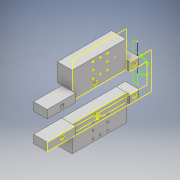
# Autodesk Inventor part: support_arret
Saved by Autodesk Inventor 2017 (Build 210142000, 142)
## iProperties
Part Number: support_arret
Material: Générique
Document SubType Name: Modeling
Designer: Thomas
Density: 1 g/cm^3
Appearance: Par défaut
Author: Thomas
Autodesk Inventor part; units mm, degrees
ref_plane "YZ Plane" through (0, 0, 0) normal (1, 0, 0) x (0, 1, 0)
ref_plane "XZ Plane" through (0, 0, 0) normal (0, 1, 0) x (-1, 0, 0)
ref_plane "XY Plane" through (0, 0, 0) normal (0, 0, 1) x (1, 0, 0)
sketch "Esquisse1" plane through (0, 0, 0) normal (1, 0, 0) x (0, 1, 0)
  line L0 (-54.8063, -40.1439) -> (54.7548, -40.1439)
  line L1 (54.7548, 0.0046) -> (-54.8063, 0.0046)
  line L2 (41.6156, -39.9954) -> (41.6156, -34.9954) construction
  line L3 (41.6156, -34.9954) -> (-43.4679, -34.9954) construction
  circle A0 centre (41.6156, -34.9954) radius 2.15
  circle A1 centre (1.6156, -34.9954) radius 2.15
  circle A2 centre (-38.3844, -34.9954) radius 2.15
  circle A3 centre (41.6156, -4.9954) radius 2.15
  circle A4 centre (1.6156, -4.9954) radius 2.15
  circle A5 centre (-38.3844, -4.9954) radius 2.15
  line L4 (-38.3844, 0.0046) -> (-38.3844, -4.9954) construction
  line L5 (54.7548, -40.1439) -> (59.7548, -40.1439)
  line L6 (59.7548, -40.1439) -> (59.7548, 0.0046)
  line L7 (59.7548, 0.0046) -> (54.7548, 0.0046)
  line L8 (-54.8063, -31.1439) -> (55.1937, -31.1439)
  line L9 (-54.8063, -8.9954) -> (55.1937, -8.9954)
  line L10 (-54.8063, 0.0046) -> (-54.8063, -8.9954)
  line L11 (-54.8063, -31.1439) -> (-54.8063, -40.1439)
  line L12 (55.1937, -31.1439) -> (55.1937, -8.9954)
  line L13 (-54.8063, -31.1439) -> (-54.8063, -40.1439)
  line L14 (-54.8063, -40.1439) -> (59.7548, -40.1439)
  line L15 (59.7548, -40.1439) -> (59.7548, 0.0046)
  line L16 (59.7548, 0.0046) -> (-54.8063, 0.0046)
  line L17 (-54.8063, 0.0046) -> (-54.8063, -8.9954)
  line L18 (-54.8063, -8.9954) -> (55.1937, -8.9954)
  line L19 (55.1937, -8.9954) -> (55.1937, -31.1439)
  line L20 (55.1937, -31.1439) -> (-54.8063, -31.1439)
  point P0 (0, 0)
  point P1 (60.2697, -11.7227)
  dimension "d4" = 5
  dimension "d5" = 4.3
  dimension "d6" = 40
  dimension "d7" = 30
  dimension "d8" = 5
  dimension "d9" = 5
  dimension "d10" = 110
  dimension "d11" = 9
  dimension "d12" = 110
  dimension "d14" = 40.1485
  dimension "d15" = 9
  constraints: 42 end point, 6 centre point, 5 collinear, 5 horizontal, 4 perpendicular, 4 vertical, 2 coincident, 2 parallel, 1 point on line, 10 other
  measures "d4" distance of L2.start L2.end
  measures "d5" diameter of A0
  measures "d6" distance of A0.centre A1.centre
  measures "d7" distance of A0.centre A3.centre
  measures "d8" distance of L4.start L4.end
  measures "d9" distance of L7.end L6.end
  measures "d10" distance of L8.start L8.end
  measures "d11" distance between parallel lines of L8 L0
  measures "d12" distance of L9.start L9.end
  measures "d14" distance between parallel lines of L1 L0
  measures "d15" distance between parallel lines of L1 L9
extrude "Extrusion1" add sketch "Esquisse1" along normal blind 15
sketch "Esquisse2" plane through (0, 59.7548, 0.0046) normal (0, 1, 0) x (1, 0, 0)
  point P0 (0, 0.0046)
sketch "Esquisse3" plane through (0, 59.7548, 0.0046) normal (0, 1, 0) x (1, 0, 0)
  line L0 (-4.433, 21.1485) -> (-2.433, 21.1485)
  arc A0 (11.3752, 24.099) -> (-2.433, 21.1485) centre (5, 20.1485) ccw
  line L1 (11.3752, 24.099) -> (12.5262, 24.099)
  arc A1 (12.5262, 24.099) -> (5, 28.6485) centre (5, 20.1485) ccw
  line L2 (5, 28.6485) -> (5, 30.0821)
  line L3 (5, 30.0821) -> (0, 30.0821)
  line L4 (0, 30.0821) -> (0, 40.1485)
  line L5 (-5.0769, 40.1485) -> (0, 40.1485)
  line L6 (-5.0769, 0.1485) -> (-5.0769, 40.1485)
  line L7 (0, 0.1485) -> (-5.0769, 0.1485)
  line L8 (0, 10.1485) -> (0, 0.1485)
  line L9 (0, 10.1485) -> (5, 10.1485)
  line L10 (5, 10.1485) -> (5, 11.6485)
  arc A2 (5, 11.6485) -> (12.5262, 16.1979) centre (5, 20.1485) ccw
  line L11 (12.5262, 16.1979) -> (11.3752, 16.1979)
  arc A3 (-2.433, 19.1485) -> (11.3752, 16.1979) centre (5, 20.1485) ccw
  line L12 (-2.433, 19.1485) -> (-4.433, 19.1485)
  line L13 (-4.433, 19.1485) -> (-4.433, 21.1485)
  line L14 (0, 0) -> (0, 9) projected
  line L15 (0, 40.1485) -> (0, 0)
  point P0 (0, 0.0046)
  point P1 (-5.0769, 30.0821)
  constraints: 30 end point, 8 point on circle, 4 centre point, 2 collinear
sketch "Esquisse4" plane through (0, 59.7548, 0.0046) normal (0, 1, 0) x (1, 0, 0)
  circle A0 centre (5.0199, 20.1961) radius 6
  circle A1 centre (5.0199, 20.1961) radius 6
  point P0 (0, 0.0046)
  dimension "d18" = 12
  constraints: 2 centre point, 1 coincident, 1 concentric
  measures "d18" diameter of A0
extrude "Extrusion2" cut sketch "Esquisse4" against normal blind 15
sketch "Esquisse5" plane through (0, -54.8063, 0.0046) normal (0, 0, 1) x (1, 0, 0)
  line L0 (15, 114.5611) -> (15, 0) construction
  line L1 (15, 114.5611) -> (11.2, 114.5611) construction
  line L2 (0, 114.5611) -> (15, 114.5611) construction
  line L3 (11.2, 114.5611) -> (11.2, 58.3541) construction
  line L4 (15, 91.0895) -> (11.2, 91.0895)
  line L5 (11.2, 91.0895) -> (11.2, 31.0895)
  line L6 (11.2, 31.0895) -> (15, 31.0895)
  line L7 (15, 31.0895) -> (15, 91.0895)
  point P0 (0, 54.8063)
  dimension "d21" = 3.8
  dimension "d22" = 60
  constraints: 12 end point, 4 perpendicular, 4 point on line, 1 collinear
  measures "d21" distance of L0.start L1.end
  measures "d22" distance of L4.end L5.end
extrude "Extrusion3" cut sketch "Esquisse5" against normal blind 15
sketch "Esquisse6" plane through (0, -54.8063, 0.0046) normal (0, 0, 1) x (1, 0, 0)
  line L0 (11.2, 91.0895) -> (11.2, 31.0895) projected
  line L1 (11.2, 91.0895) -> (-5, 91.0895)
  line L2 (-5, 91.0895) -> (-5, 31.3621)
  line L3 (-5, 31.3621) -> (11.2, 31.3621)
  line L4 (11.2, 31.3621) -> (11.2, 91.0895)
  point P0 (0, 54.8063)
  dimension "d25" = 16.2
  constraints: 8 end point, 2 parallel, 1 horizontal, 1 perpendicular
  measures "d25" distance of L3.end L2.end
extrude "Extrusion4" add sketch "Esquisse6" along normal blind 30
sketch "Esquisse7" plane through (11.2, -23.7168, -8.9954) normal (1, 0, 0) x (0, 0, -1)
  line L0 (0, 60) -> (0, 0) projected
  line L1 (-9, 60) -> (0, 60) projected
  line L2 (-9, 60) -> (-39, 60) projected
  line L3 (-39, 0.2726) -> (-39, 60) projected
  line L4 (-9, 0.2726) -> (-39, 0.2726) projected
  line L5 (-9, 0) -> (-9, 0.2726) projected
  line L6 (-9, 0) -> (0, 0) projected
  circle A0 centre (-4, 25.3324) radius 2.15 projected
  circle A1 centre (-10, 31.1304) radius 1
  circle A2 centre (-18, 39.1304) radius 1
  circle A3 centre (-26, 39.1304) radius 1
  circle A4 centre (-26, 31.1304) radius 1
  circle A5 centre (-26, 23.1304) radius 1
  circle A6 centre (-18, 23.1304) radius 1
  circle A7 centre (-10, 23.1304) radius 1
  circle A8 centre (-10, 39.1304) radius 1
  point P0 (-8.9954, 23.7168)
  dimension "d28" = 10
  dimension "d29" = 16
  dimension "d30" = 8
  dimension "d31" = 8
  dimension "d32" = 8
  dimension "d33" = 8
  dimension "d34" = 8
  dimension "d35" = 8
  constraints: 8 centre point
  measures "d28" distance from line of L0 A1.centre
  measures "d29" distance of A4.centre A1.centre
  measures "d30" distance of A7.centre A1.centre
  measures "d31" distance of A8.centre A1.centre
  measures "d32" distance of A6.centre A7.centre
  measures "d33" distance of A5.centre A6.centre
  measures "d34" distance of A2.centre A8.centre
  measures "d35" distance of A3.centre A2.centre
extrude "Extrusion5" cut sketch "Esquisse7" against normal blind 30 contours A1 | A2 | A3 | A4 | A5 | A6 | A7 | A8
sketch "Esquisse8" plane through (15, 0, 0) normal (1, 0, 0) x (0, 0, -1)
  line L0 (-0.0046, 36.2832) -> (8.9954, 36.2832) projected
  line L1 (8.9954, 36.2832) -> (8.9954, 55.1937) projected
  line L2 (8.9954, 55.1937) -> (31.1439, 55.1937) projected
  line L3 (31.1439, 55.1937) -> (31.1439, -54.8063) projected
  line L4 (31.1439, -54.8063) -> (40.1439, -54.8063) projected
  line L5 (40.1439, -54.8063) -> (40.1439, 59.7548) projected
  line L6 (40.1439, 59.7548) -> (-0.0046, 59.7548) projected
  line L7 (-0.0046, 59.7548) -> (-0.0046, 36.2832) projected
  circle A0 centre (4.9954, 41.6156) radius 2.15 projected
  circle A1 centre (34.9954, -38.3844) radius 2.15 projected
  circle A2 centre (34.9954, 1.6156) radius 2.15 projected
  circle A3 centre (34.9954, 41.6156) radius 2.15 projected
  point P0 (0, 0)
sketch "Esquisse9" plane through (11.2, -23.7168, -8.9954) normal (1, 0, 0) x (0, 0, -1)
  circle A0 centre (-10, 23.1304) radius 1 projected
  circle A1 centre (-26, 23.1304) radius 1 projected
  circle A2 centre (-26, 39.1304) radius 1 projected
  circle A3 centre (-10, 31.1304) radius 1 projected
  circle A4 centre (-18, 39.1304) radius 1 projected
  circle A5 centre (-26, 31.1304) radius 1 projected
  circle A6 centre (-18, 23.1304) radius 1 projected
  circle A7 centre (-10, 39.1304) radius 1 projected
  line L0 (0, 60) -> (0, 0) projected
  line L1 (-9, 60) -> (0, 60) projected
  line L2 (-9, 60) -> (-39, 60) projected
  line L3 (-39, 0.2726) -> (-39, 60) projected
  line L4 (-9, 0.2726) -> (-39, 0.2726) projected
  line L5 (-9, 0) -> (-9, 0.2726) projected
  line L6 (-9, 0) -> (0, 0) projected
  circle A8 centre (-4, 25.3324) radius 2.15 projected
  point P0 (-8.9954, 23.7168)
sketch "Esquisse10" plane through (15, 0, 0) normal (1, 0, 0) x (0, 0, -1)
  line L0 (31.0084, 36.2646) -> (31.0084, -23.7354)
  circle A0 centre (41.0084, -0.605) radius 1
  circle A1 centre (57.0084, -0.605) radius 1
  circle A2 centre (57.0084, 15.395) radius 1
  circle A3 centre (41.0084, 7.395) radius 1
  circle A4 centre (49.0084, 15.395) radius 1
  circle A5 centre (57.0084, 7.395) radius 1
  circle A6 centre (49.0084, -0.605) radius 1
  circle A7 centre (41.0084, 15.395) radius 1
  line L1 (40.0084, 36.2646) -> (31.0084, 36.2646)
  line L2 (40.0084, 36.2646) -> (70.0084, 36.2646)
  line L3 (70.0084, -23.4628) -> (70.0084, 36.2646)
  line L4 (40.0084, -23.4628) -> (70.0084, -23.4628)
  line L5 (40.0084, -23.7354) -> (40.0084, -23.4628)
  line L6 (40.0084, -23.7354) -> (31.0084, -23.7354)
  circle A8 centre (35.0084, 1.597) radius 2.15
  point P0 (0, 0)
  point P1 (40.0039, -0.0185)
  constraints: 14 end point, 9 centre point
extrude "Extrusion6" cut sketch "Esquisse10" against normal blind 3.8 contours L1 L2 L3 L4 L5 L6 L0 | A0 | A1 | A2 | A3 | A4 | A5 | A6 | A7 | A8
sketch "Esquisse11" plane through (11.2, 0, 0) normal (1, 0, 0) x (0, 0, -1)
  circle A0 centre (34.9954, 1.6156) radius 2.15 projected
  line L0 (31.1439, -23.7354) -> (31.1439, 36.2646) projected
  line L1 (40.0084, -23.7354) -> (31.1439, -23.7354) projected
  line L2 (40.0084, -23.4628) -> (40.0084, -23.7354) projected
  line L3 (40.1439, -23.4628) -> (40.0084, -23.4628) projected
  line L4 (40.1439, 36.2646) -> (40.1439, -23.4628) projected
  line L5 (31.1439, 36.2646) -> (40.1439, 36.2646) projected
  point P0 (0, 0)
sketch "Esquisse12" plane through (11.2, 0, 0) normal (1, 0, 0) x (0, 0, -1)
  point P0 (-8.9954, 23.7168)
sketch "Esquisse13" plane through (11.2, 0, 0) normal (1, 0, 0) x (0, 0, -1)
  line L0 (30.9931, 36.2812) -> (30.9931, -23.7188)
  circle A0 centre (40.9931, -0.5884) radius 1
  circle A1 centre (56.9931, -0.5884) radius 1
  circle A2 centre (56.9931, 15.4116) radius 1
  circle A3 centre (40.9931, 7.4116) radius 1
  circle A4 centre (48.9931, 15.4116) radius 1
  circle A5 centre (56.9931, 7.4116) radius 1
  circle A6 centre (48.9931, -0.5884) radius 1
  circle A7 centre (40.9931, 15.4116) radius 1
  line L1 (39.9931, 36.2812) -> (30.9931, 36.2812)
  line L2 (39.9931, 36.2812) -> (69.9931, 36.2812)
  line L3 (69.9931, -23.4462) -> (69.9931, 36.2812)
  line L4 (39.9931, -23.4462) -> (69.9931, -23.4462)
  line L5 (39.9931, -23.7188) -> (39.9931, -23.4462)
  line L6 (39.9931, -23.7188) -> (30.9931, -23.7188)
  circle A8 centre (34.9931, 1.6136) radius 2.15
  point P0 (0, 0)
  point P1 (39.9885, -0.002)
  constraints: 14 end point, 9 centre point
extrude "Extrusion7" add sketch "Esquisse13" against normal blind 16.2
sketch "Esquisse14" plane through (-5, 0, 0) normal (-1, 0, 0) x (0, 0, 1)
  circle A0 centre (-56.9931, -0.5884) radius 1 projected
  circle A1 centre (-56.9931, 7.4116) radius 1 projected
  circle A2 centre (-56.9931, 15.4116) radius 1 projected
  circle A3 centre (-48.9931, 15.4116) radius 1 projected
  circle A4 centre (-48.9931, -0.5884) radius 1 projected
  circle A5 centre (-40.9931, -0.5884) radius 1 projected
  circle A6 centre (-40.9931, 7.4116) radius 1 projected
  circle A7 centre (-40.9931, 15.4116) radius 1 projected
  circle A8 centre (-56.9931, -0.5884) radius 1 projected
  circle A9 centre (-56.9931, -0.5884) radius 3
  line L0 (-56.9931, -0.5884) -> (-56.9931, 15.4116) construction
  line L1 (-56.9931, 15.4116) -> (-40.9931, 15.4116) construction
  circle A10 centre (-56.9931, 7.4116) radius 3
  circle A11 centre (-56.9931, 15.4116) radius 3
  circle A12 centre (-48.9931, -0.5884) radius 3
  circle A13 centre (-48.9931, 7.4116) radius 3
  circle A14 centre (-48.9931, 15.4116) radius 3
  circle A15 centre (-40.9931, -0.5884) radius 3
  circle A16 centre (-40.9931, 7.4116) radius 3
  circle A17 centre (-40.9931, 15.4116) radius 3
  line L2 (-26.1915, 59.7548) -> (-14.1915, 59.7548) construction
  line L3 (-20.1915, 59.7548) -> (-20.1915, -51.3949) construction
  circle A18 centre (16.6101, -0.5884) radius 1
  circle A19 centre (16.6101, 7.4116) radius 1
  circle A20 centre (16.6101, 15.4116) radius 1
  circle A21 centre (8.6101, 15.4116) radius 1
  circle A22 centre (8.6101, -0.5884) radius 1
  circle A23 centre (0.6101, -0.5884) radius 1
  circle A24 centre (0.6101, 7.4116) radius 1
  circle A25 centre (0.6101, 15.4116) radius 1
  circle A26 centre (16.6101, -0.5884) radius 1
  circle A27 centre (16.6101, -0.5884) radius 3
  line L4 (16.6101, -0.5884) -> (16.6101, 15.4116) construction
  line L5 (16.6101, 15.4116) -> (0.6101, 15.4116) construction
  circle A28 centre (16.6101, 7.4116) radius 3
  circle A29 centre (16.6101, 15.4116) radius 3
  circle A30 centre (8.6101, -0.5884) radius 3
  circle A31 centre (8.6101, 7.4116) radius 3
  circle A32 centre (8.6101, 15.4116) radius 3
  circle A33 centre (0.6101, -0.5884) radius 3
  circle A34 centre (0.6101, 7.4116) radius 3
  circle A35 centre (0.6101, 15.4116) radius 3
  point P0 (0, 0)
  point P1 (-23.478, 59.7548)
  point P2 (-16.9051, 59.7548)
  dimension "d44" = 6
  dimension "d47" = 8
  dimension "d50" = 8
  constraints: 27 centre point, 18 symmetric about line, 10 end point, 3 vertical, 2 coincident, 1 horizontal, 1 midpoint, 1 perpendicular, 34 other
  measures "d44" diameter of A9
  measures "d47" distance of A9.centre A10.centre
  measures "d50" distance of A9.centre A12.centre
extrude "Extrusion8" cut sketch "Esquisse14" against normal blind 8 contours A0 | A1 | A2 | A3 | A4 | A5 | A6 | A7 | A9 | A10 | A11 | A12 | A14 | A15 | A16 | A17 | A18 | A19 | A20 | A21 | A22 | A23 | A24 | A25 | A27 | A28 | A29 | A30 | A32 | A33 | A34 | A35
sketch "Esquisse15" plane through (-5, 0, 0) normal (-1, 0, 0) x (0, 0, 1)
  line L0 (-39.9931, -23.7188) -> (-30.9931, -23.7188) projected
  line L1 (-40.1439, 36.2646) -> (-40.1439, 59.7548) projected
  line L2 (-30.9931, -23.7188) -> (-40.1439, -23.7188)
  line L3 (-40.1439, -23.7188) -> (-40.1439, 36.2646)
  line L4 (-40.1439, 36.2646) -> (-30.9931, 36.2646)
  line L5 (-30.9931, 36.2646) -> (-30.9931, -23.7188)
  line L6 (-40.1439, 36.2646) -> (-30.9931, 36.2646)
  line L7 (-30.9931, 36.2646) -> (-30.9931, 36.6984)
  line L8 (-30.9931, 36.6984) -> (-40.1439, 36.6984)
  line L9 (-40.1439, 36.6984) -> (-40.1439, 36.2646)
  point P0 (0, 0)
  constraints: 16 end point, 4 parallel, 2 horizontal, 2 perpendicular
extrude "Extrusion9" cut sketch "Esquisse15" against normal blind 5
sketch "Esquisse16" plane through (11.2, -23.7188, -30.9931) normal (0, 0, 1) x (1, 0, 0)
  line L0 (-11.2, 60) -> (-11.2, 0) projected
  line L1 (0, 0) -> (-11.2, 0) projected
  line L2 (0, 0) -> (0, 60) projected
  line L3 (0, 60) -> (-11.2, 60) projected
  point P0 (-11.2, 23.7188)
extrude "Extrusion10" cut sketch "Esquisse16" against normal blind 0.15
sketch "Esquisse17" plane through (11.2, 0, 0) normal (1, 0, 0) x (0, 0, -1)
  line L0 (31.1431, 36.2812) -> (31.1431, -23.7188) projected
  line L1 (31.1439, -23.7188) -> (31.1431, -23.7188) projected
  line L2 (31.1439, -23.7354) -> (31.1439, -23.7188) projected
  line L3 (40.0084, -23.7354) -> (31.1439, -23.7354) projected
  line L4 (40.0084, -23.4628) -> (40.0084, -23.7354) projected
  line L5 (40.1439, -23.4628) -> (40.0084, -23.4628) projected
  line L6 (40.1439, -23.4462) -> (40.1439, -23.4628) projected
  line L7 (69.9931, -23.4462) -> (40.1439, -23.4462) projected
  line L8 (69.9931, 36.2812) -> (69.9931, -23.4462) projected
  line L9 (40.1439, 36.2812) -> (69.9931, 36.2812) projected
  line L10 (40.1439, 36.2646) -> (40.1439, 36.2812) projected
  line L11 (31.1439, 36.2646) -> (40.1439, 36.2646) projected
  line L12 (31.1439, 36.2812) -> (31.1439, 36.2646) projected
  line L13 (31.1431, 36.2812) -> (31.1439, 36.2812) projected
  line L14 (40.1439, -0.0603) -> (40.1439, -1.1165) projected
  arc A0 (40.1439, -1.1165) -> (40.1439, -0.0603) centre (40.9931, -0.5884) ccw projected
  line L15 (40.1439, 7.9397) -> (40.1439, 6.8835) projected
  arc A1 (40.1439, 6.8835) -> (40.1439, 7.9397) centre (40.9931, 7.4116) ccw projected
  line L16 (40.1439, 15.9397) -> (40.1439, 14.8835) projected
  arc A2 (40.1439, 14.8835) -> (40.1439, 15.9397) centre (40.9931, 15.4116) ccw projected
  circle A3 centre (48.9931, -0.5884) radius 1 projected
  circle A4 centre (56.9931, -0.5884) radius 1 projected
  circle A5 centre (56.9931, 7.4116) radius 1 projected
  circle A6 centre (48.9931, 15.4116) radius 1 projected
  circle A7 centre (56.9931, 15.4116) radius 1 projected
  arc A8 (33.6113, 3.2608) -> (36.3772, -0.0316) centre (34.9954, 1.6156) ccw projected
  arc A9 (36.3772, -0.0316) -> (33.6113, 3.2608) centre (34.9931, 1.6136) ccw projected
  line L17 (69.9931, -23.4462) -> (40.1439, -23.4462) projected
  line L18 (59.9931, -23.4462) -> (59.9931, 36.2812)
  line L19 (40.1439, 36.2812) -> (69.9931, 36.2812) projected
  line L20 (26.1915, 55.1937) -> (14.1915, 55.1937) construction
  line L21 (20.1915, 55.1937) -> (20.1915, -54.679) construction
  line L22 (-19.6101, -23.4462) -> (-19.6101, 36.2812)
  circle A10 centre (-1.0046, -0.5864) radius 1 projected
  circle A11 centre (-17.0046, -0.5864) radius 1 projected
  circle A12 centre (-17.0046, 15.4136) radius 1 projected
  circle A13 centre (-1.0046, 7.4136) radius 1 projected
  circle A14 centre (-9.0046, 15.4136) radius 1 projected
  circle A15 centre (-17.0046, 7.4136) radius 1 projected
  circle A16 centre (-9.0046, -0.5864) radius 1 projected
  circle A17 centre (-1.0046, 15.4136) radius 1 projected
  line L23 (8.9954, 36.2832) -> (8.9954, -23.7168) projected
  line L24 (-0.0046, 36.2832) -> (8.9954, 36.2832) projected
  line L25 (-0.0046, 36.2832) -> (-30.0046, 36.2832) projected
  line L26 (-30.0046, -23.4442) -> (-30.0046, 36.2832) projected
  line L27 (-0.0046, -23.4442) -> (-30.0046, -23.4442) projected
  line L28 (-0.0046, -23.7168) -> (-0.0046, -23.4442) projected
  line L29 (-0.0046, -23.7168) -> (8.9954, -23.7168) projected
  circle A18 centre (4.9954, 1.6156) radius 2.15 projected
  line L30 (-19.6101, -23.4462) -> (-19.6101, 36.2812)
  line L31 (-0.0046, 36.2832) -> (-30.0046, 36.2832) projected
  point P0 (0, 0)
  point P1 (16.9051, 55.1937)
  point P2 (23.478, 55.1937)
  dimension "d59" = 10
  constraints: 8 end point, 2 point on line, 2 symmetric about line, 2 vertical, 1 midpoint, 1 perpendicular
  measures "d59" distance between parallel lines of L18 L8
extrude "Extrusion11" cut sketch "Esquisse17" against normal blind 52.35 contours L9 L8 L7 L18
sketch "Esquisse18" plane through (11.2, -23.7168, -8.9954) normal (1, 0, 0) x (0, 0, -1)
  circle A0 centre (-10, 23.1304) radius 1 projected
  circle A1 centre (-26, 23.1304) radius 1 projected
  circle A2 centre (-26, 39.1304) radius 1 projected
  circle A3 centre (-10, 31.1304) radius 1 projected
  circle A4 centre (-18, 39.1304) radius 1 projected
  circle A5 centre (-26, 31.1304) radius 1 projected
  circle A6 centre (-18, 23.1304) radius 1 projected
  circle A7 centre (-10, 39.1304) radius 1 projected
  line L0 (0, 60) -> (0, 0) projected
  line L1 (-9, 60) -> (0, 60) projected
  line L2 (-9, 60) -> (-39, 60) projected
  line L3 (-39, 0.2726) -> (-39, 60) projected
  line L4 (-9, 0.2726) -> (-39, 0.2726) projected
  line L5 (-9, 0) -> (-9, 0.2726) projected
  line L6 (-9, 0) -> (0, 0) projected
  circle A8 centre (-4, 25.3324) radius 2.15 projected
  line L7 (-9, 0.2726) -> (-39, 0.2726) projected
  line L8 (-29, 0.2726) -> (-29, 60)
  line L9 (-9, 60) -> (-39, 60) projected
  line L10 (-39, 0.2726) -> (-39, 60) projected
  line L11 (-29, 0.2726) -> (-39, 0.2726)
  line L12 (-39, 0.2726) -> (-39, 60)
  line L13 (-39, 60) -> (-29, 60)
  line L14 (-29, 60) -> (-29, 0.2726)
  point P0 (-8.9954, 23.7168)
  dimension "d62" = 10
  constraints: 10 end point, 2 parallel, 2 perpendicular, 2 point on line, 1 horizontal
  measures "d62" distance between parallel lines of L3 L8
extrude "Extrusion12" cut sketch "Esquisse18" against normal blind 41.15 contours L8 L4 L3 L2
sketch "Esquisse19" plane through (15, 0, 0) normal (1, 0, 0) x (0, 0, -1)
  line L0 (-5.813, 46.3829) -> (44.8085, 46.3829)
  line L1 (44.8085, 46.3829) -> (44.8085, 65.2751)
  line L2 (44.8085, 65.2751) -> (-5.813, 65.2751)
  line L3 (-5.813, 65.2751) -> (-5.813, 46.3829)
  point P0 (0, 0)
  constraints: 8 end point, 2 parallel, 1 horizontal, 1 perpendicular
extrude "Extrusion13" cut sketch "Esquisse19" against normal blind 19
